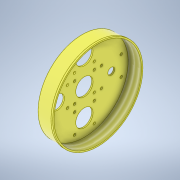
# Autodesk Inventor part: Container_Lid(Sunpet_2L)
Saved by Autodesk Inventor 2020 (Build 240168000, 168)
## iProperties
Created: 2021-04-27
Part Number: Container_Lid(Sunpet_2L)
Material: Generic
Document SubType Name: Modeling
Designer: Workshop
Density: 1 g/cm^3
Appearance: Smooth - Yellow
Author: Workshop
Autodesk Inventor part; units mm, degrees
ref_plane "YZ Plane" through (0, 0, 0) normal (1, 0, 0) x (0, 1, 0)
ref_plane "XZ Plane" through (0, 0, 0) normal (0, 1, 0) x (-1, 0, 0)
ref_plane "XY Plane" through (0, 0, 0) normal (0, 0, 1) x (1, 0, 0)
sketch "Sketch1" plane through (0, 0, 0) normal (0, 0, 1) x (1, 0, 0)
  line L0 (0, 0) -> (0, -47.625)
  line L1 (0, -47.625) -> (-1, -47.625)
  line L2 (-1, -47.625) -> (-1, -50.875)
  line L3 (14.9886, -51.478) -> (14.9831, -51.978)
  line L4 (14.9831, -51.978) -> (16.983, -52)
  line L5 (16.983, -52) -> (16.9995, -50.5001)
  line L6 (16.9995, -50.5001) -> (1.5, -50.5001)
  line L7 (1.5, -50.5001) -> (1.5, 0)
  line L8 (1.5, 0) -> (0, 0)
  line L9 (-4.5999, 0) -> (20.5994, 0) projected
  line L10 (-1, -50.875) -> (14.9886, -51.478)
  dimension "d0" = 1.5
  dimension "d1" = 2
  dimension "d2" = 0.5
  dimension "d3" = 16
  dimension "d4" = 3.25
  dimension "d5" = 1
  dimension "d6" = 1.5
  dimension "d10" = 50.875
  dimension "d11" = 15.4995
  dimension "d17" = 52
  constraints: 20 end point, 5 perpendicular, 1 horizontal, 1 vertical
  measures "d0" distance of L4.end L5.end
  measures "d1" distance of L3.end L4.end
  measures "d2" distance of L3.start L3.end
  measures "d3" distance of L2.end L3.start
  measures "d4" distance of L1.end L2.end
  measures "d5" distance of L0.end L1.end
  measures "d6" distance between parallel lines of L0 L7
  measures "d10" vertical distance of L0.start L2.end
  measures "d11" distance of L5.end L6.end
  measures "d17" distance from line of L9 L4.end
revolve "Revolution1" add sketch "Sketch1" angle 360 about axis through (-10, 0, 0) along (1, 0, 0)
thread "Thread1" size "M100x6" class "6H" standard "ANSI Metric M Profile" full length
sketch "Sketch4" plane through (0, 0, 0) normal (-1, 0, 0) x (0, 0, 1)
  point P0 (0, 0)
  point P1 (0, 0)
  constraints: 1 coincident
sketch "Sketch5" plane through (0, 0, 0) normal (-1, 0, 0) x (0, 0, 1)
  circle A0 centre (-11.4021, -42.3779) radius 1.5 projected
  circle A1 centre (-11.4021, -19.5737) radius 1.5 projected
  circle A2 centre (11.4021, -19.5736) radius 1.5 projected
  circle A3 centre (11.4021, -42.3778) radius 1.5 projected
  circle A4 centre (0, -30.9758) radius 10 projected
  circle A5 centre (-42.3779, 11.4021) radius 1.5 projected
  circle A6 centre (-19.5737, 11.4021) radius 1.5 projected
  circle A7 centre (-19.5736, -11.4021) radius 1.5 projected
  circle A8 centre (-42.3778, -11.4021) radius 1.5 projected
  circle A9 centre (11.4021, 42.3779) radius 1.5 projected
  circle A10 centre (11.4021, 19.5737) radius 1.5 projected
  circle A11 centre (-11.4021, 19.5736) radius 1.5 projected
  circle A12 centre (-11.4021, 42.3778) radius 1.5 projected
  circle A13 centre (0, 30.9758) radius 10 projected
  circle A14 centre (42.3779, -11.4021) radius 1.5 projected
  circle A15 centre (19.5737, -11.4021) radius 1.5 projected
  circle A16 centre (19.5736, 11.4021) radius 1.5 projected
  circle A17 centre (42.3778, 11.4021) radius 1.5 projected
  circle A18 centre (11.4021, -11.4021) radius 1.5 projected
  circle A19 centre (-11.4021, -11.4021) radius 1.5 projected
  circle A20 centre (-11.4021, 11.4021) radius 1.5 projected
  circle A21 centre (11.4021, 11.4021) radius 1.5 projected
  circle A22 centre (30.9758, 0) radius 8 projected
  circle A23 centre (0, 0) radius 10 projected
extrude "Extrusion3" cut sketch "Sketch5" against normal through all
sketch "Sketch6" plane through (0, 0, 0) normal (-1, 0, 0) x (0, 0, 1)
  circle A0 centre (-30.9758, 0) radius 4
  circle A1 centre (-19.5736, -11.4021) radius 1.5 projected
  circle A2 centre (-19.5737, 11.4021) radius 1.5 projected
  point P0 (0, 0)
  dimension "d24" = 8
  dimension "d25" = 16.125
  constraints: 1 centre point, 1 horizontal alignment
  measures "d24" diameter of A0
  measures "d25" distance of A1.centre A0.centre
extrude "Extrusion4" cut sketch "Sketch6" against normal through all contours A0
body "Solid1"
